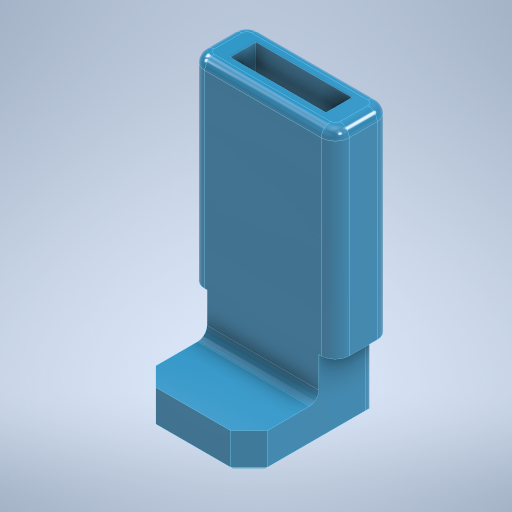
# Autodesk Inventor part: BaseAux_Sensor
Saved by Autodesk Inventor 2024 (Build 280153000, 153)
## iProperties
Created: 2023-11-04
Part Number: BaseAux_Sensor
Material: Generic
Document SubType Name: Modeling
Designer: fredy
Density: 1 g/cm^3
Appearance: Sky Blue Dark
Author: fredy
Autodesk Inventor part; units mm, degrees
ref_plane "YZ Plane" through (0, 0, 0) normal (1, 0, 0) x (0, 1, 0)
ref_plane "XZ Plane" through (0, 0, 0) normal (0, 1, 0) x (-1, 0, 0)
ref_plane "XY Plane" through (0, 0, 0) normal (0, 0, 1) x (1, 0, 0)
sketch "Sketch5" plane through (0, 0, 0) normal (0, 0, 1) x (1, 0, 0)
  line L0 (0, 0) -> (31, 0)
  line L1 (31, 0) -> (31, 58.9)
  line L2 (31, 58.9) -> (0, 58.9)
  line L3 (0, 58.9) -> (0, 0)
  dimension "d33" = 31
  constraints: 8 end point, 2 parallel, 1 horizontal, 1 perpendicular
  measures "d33" distance of L1.end L2.end
extrude "Extrusion5" add sketch "Sketch5" along normal blind 12
sketch "Sketch6" plane through (0, 0, 12) normal (0, 0, 1) x (1, 0, 0)
  line L0 (0, 58.9) -> (0, 0) projected
  line L1 (0, 0) -> (3.5, 0)
  line L2 (3.5, 0) -> (3.5, 16.4)
  line L3 (3.5, 16.4) -> (0, 16.4)
  line L4 (0, 16.4) -> (0, 0)
  line L5 (0, 0) -> (31, 0) projected
  line L6 (31, 0) -> (27.5, 0)
  line L7 (27.5, 0) -> (27.5, 16.4)
  line L8 (27.5, 16.4) -> (31, 16.4)
  line L9 (31, 16.4) -> (31, 0)
  dimension "d40" = 24
  dimension "d41" = 16.4
  constraints: 16 end point, 4 parallel, 2 equal length, 2 horizontal, 2 perpendicular
  measures "d40" distance between parallel lines of L7 L2
  measures "d41" distance of L1.end L2.end
extrude "Extrusion6" cut sketch "Sketch6" against normal up to surface (12 mm away)
sketch "Sketch7" plane through (0, 0, 12) normal (0, 0, 1) x (1, 0, 0)
  line L0 (3.5, 0) -> (27.5, 0) projected
  line L1 (3.5, 0) -> (27.5, 0)
  line L2 (27.5, 0) -> (27.5, 7.8)
  line L3 (27.5, 7.8) -> (3.5, 7.8)
  line L4 (3.5, 7.8) -> (3.5, 0)
  point P0 (0, 0)
  dimension "d44" = 7.8
  constraints: 8 end point, 2 parallel, 1 horizontal, 1 perpendicular
  measures "d44" distance of L3.end L0.start
extrude "Extrusion7" add sketch "Sketch7" along normal blind 15
sketch "Sketch8" plane through (0, 58.9, 0) normal (0, 1, 0) x (1, 0, 0)
  line L0 (31, -12) -> (0, -12) projected
  line L1 (31, 0) -> (31, -12) projected
  line L2 (5.2, -8.8) -> (25.8, -8.8)
  line L3 (25.8, -8.8) -> (25.8, -3.2)
  line L4 (25.8, -3.2) -> (5.2, -3.2)
  line L5 (5.2, -3.2) -> (5.2, -8.8)
  line L6 (5.2, -8.8) -> (25.8, -3.2) construction
  line L7 (25.8, -8.8) -> (5.2, -3.2) construction
  point P0 (0, 0)
  point P1 (15.5, -6)
  point P2 (15.5, -12)
  point P3 (31, -6)
  dimension "d47" = 20.6
  dimension "d48" = 5.6
  constraints: 12 end point, 4 midpoint, 2 parallel, 1 horizontal, 1 horizontal alignment, 1 perpendicular, 1 vertical alignment
  measures "d47" distance of L3.end L4.end
  measures "d48" distance of L4.end L2.start
extrude "Extrusion8" cut sketch "Sketch8" against normal blind 17
chamfer "Chamfer3" distance 4 angle 45 2 edges at (3.5, 3.9, 27) (27.5, 3.9, 27)
chamfer "Chamfer4" distance 1 angle 45 6 edges at (3.5, 0, 11.5) (5.5, 0, 25) (15.5, 0, 27) (25.5, 0, 25) (27.5, 0, 11.5) (15.5, 0, 0)
fillet "Fillet2" radius 2 1 edges at (15.5, 7.8, 12)
fillet "Fillet3" radius 3 4 edges at (0, 37.65, 12) (31, 37.65, 12) (31, 37.65, 0) (0, 37.65, 0)
fillet "Fillet4" radius 2 8 edges at (0, 58.9, 6) (0.8787, 58.9, 0.8787) (15.5, 58.9, 0) (30.1213, 58.9, 0.8787) (31, 58.9, 6) (30.1213, 58.9, 11.1213) (15.5, 58.9, 12) (0.8787, 58.9, 11.1213)
fillet "Fillet5" radius 2 2 edges at (27.5, 8.7, 0) (3.5, 8.7, 0)
body "Solid3"
